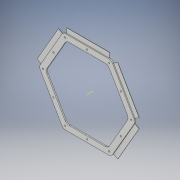
# Autodesk Inventor part: Flat Placeholder v1 - 175 - 12mm rim
Saved by Autodesk Inventor 2019 (Build 230136000, 136)
## iProperties
Created: 2021-07-14
Part Number: Flat Placeholder v1 - 175 - 12mm rim
Material: Generic
Document SubType Name: Modeling
Designer: Lix
Density: 1 g/cm^3
Appearance: Default
Author: Lix
Autodesk Inventor part; units mm, degrees
ref_plane "YZ Plane" through (0, 0, 0) normal (1, 0, 0) x (0, 1, 0)
ref_plane "XZ Plane" through (0, 0, 0) normal (0, 1, 0) x (-1, 0, 0)
ref_plane "XY Plane" through (0, 0, 0) normal (0, 0, 1) x (1, 0, 0)
sketch "Sketch1" plane through (0, 0, 0) normal (0, 0, 1) x (1, 0, 0)
  line L0 (50.5181, -87.5) -> (-50.5181, -87.5)
  line L1 (-50.5181, -87.5) -> (-101.0363, 0)
  line L2 (-101.0363, 0) -> (-50.5181, 87.5)
  line L3 (-50.5181, 87.5) -> (50.5181, 87.5)
  line L4 (50.5181, 87.5) -> (101.0363, 0)
  line L5 (101.0363, 0) -> (50.5181, -87.5)
  point P0 (0, 0)
  point P1 (0, 0)
  dimension "d0" = 175
  constraints: 12 end point, 1 coincident, 1 horizontal, 13 other
  measures "d0" distance between parallel lines of L4 L1
extrude "Extrusion1" add sketch "Sketch1" along normal blind 2
sketch "Sketch7" plane through (0, 0, 2) normal (0, 0, 1) x (1, 0, 0)
  line L0 (-50.5181, -87.5) -> (50.5181, -87.5) projected
  line L1 (50.5181, -87.5) -> (101.0363, 0) projected
  line L2 (101.0363, 0) -> (50.5181, 87.5) projected
  line L3 (50.5181, 87.5) -> (-50.5181, 87.5) projected
  line L4 (-50.5181, 87.5) -> (-101.0363, 0) projected
  line L5 (-101.0363, 0) -> (-50.5181, -87.5) projected
  line L6 (-43.5899, 75.5) -> (43.5899, 75.5)
  line L7 (43.5899, 75.5) -> (87.1799, 0)
  line L8 (87.1799, 0) -> (43.5899, -75.5)
  line L9 (43.5899, -75.5) -> (-43.5899, -75.5)
  line L10 (-43.5899, -75.5) -> (-87.1799, 0)
  line L11 (-87.1799, 0) -> (-43.5899, 75.5)
  dimension "d26" = 12
  constraints: 12 end point, 5 other
  measures "d26" distance between parallel lines of L3 L6
extrude "Extrusion6" cut sketch "Sketch7" against normal blind 7 contours L6 L7 L8 L9 L10 L11
fillet "Fillet2" radius 10 6 edges at (-87.1799, 0, 1) (-43.5899, -75.5, 1) (43.5899, -75.5, 1) (87.1799, 0, 1) (43.5899, 75.5, 1) (-43.5899, 75.5, 1)
fillet "Fillet3" radius 10 6 edges at (-50.5181, 87.5, 1) (50.5181, 87.5, 1) (101.0363, 0, 1) (50.5181, -87.5, 1) (-50.5181, -87.5, 1) (-101.0363, 0, 1)
sketch "Sketch8" plane through (0, 0, 0) normal (0, 0, -1) x (-1, 0, 0)
  line L0 (46.4767, 70.5) -> (84.2931, 5) projected
  arc A0 (84.2931, -5) -> (84.2931, 5) centre (75.6329, 0) ccw projected
  line L1 (84.2931, -5) -> (46.4767, -70.5) projected
  arc A1 (37.8164, -75.5) -> (46.4767, -70.5) centre (37.8164, -65.5) ccw projected
  line L2 (37.8164, -75.5) -> (-37.8164, -75.5) projected
  arc A2 (-46.4767, -70.5) -> (-37.8164, -75.5) centre (-37.8164, -65.5) ccw projected
  line L3 (-46.4767, -70.5) -> (-84.2931, -5) projected
  arc A3 (-84.2931, 5) -> (-84.2931, -5) centre (-75.6329, 0) ccw projected
  line L4 (-84.2931, 5) -> (-46.4767, 70.5) projected
  arc A4 (-37.8164, 75.5) -> (-46.4767, 70.5) centre (-37.8164, 65.5) ccw projected
  line L5 (-37.8164, 75.5) -> (37.8164, 75.5) projected
  arc A5 (46.4767, 70.5) -> (37.8164, 75.5) centre (37.8164, 65.5) ccw projected
  arc A6 (98.1495, -5) -> (98.1495, 5) centre (89.4893, 0) ccw projected
  line L6 (98.1495, 5) -> (53.4049, 82.5) projected
  arc A7 (53.4049, 82.5) -> (44.7446, 87.5) centre (44.7446, 77.5) ccw projected
  line L7 (44.7446, 87.5) -> (-44.7446, 87.5) projected
  arc A8 (-44.7446, 87.5) -> (-53.4049, 82.5) centre (-44.7446, 77.5) ccw projected
  line L8 (-53.4049, 82.5) -> (-98.1495, 5) projected
  arc A9 (-98.1495, 5) -> (-98.1495, -5) centre (-89.4893, 0) ccw projected
  line L9 (-98.1495, -5) -> (-53.4049, -82.5) projected
  arc A10 (-53.4049, -82.5) -> (-44.7446, -87.5) centre (-44.7446, -77.5) ccw projected
  line L10 (-44.7446, -87.5) -> (44.7446, -87.5) projected
  arc A11 (44.7446, -87.5) -> (53.4049, -82.5) centre (44.7446, -77.5) ccw projected
  line L11 (53.4049, -82.5) -> (98.1495, -5) projected
  line L12 (-53.4049, -82.5) -> (-62.0652, -87.5)
  line L13 (-62.0652, -87.5) -> (-106.8098, -10)
  line L14 (-53.4049, -82.5) -> (-98.1495, -5) projected
  line L15 (-106.8098, -10) -> (-98.1495, -5)
  line L16 (-98.1495, -5) -> (-53.4049, -82.5) projected
  line L17 (-53.4049, -82.5) -> (-98.1495, -5)
  point P0 (0, 0)
  point P1 (0, 0)
  dimension "d27" = 10
  constraints: 8 end point, 2 parallel, 2 perpendicular, 1 coincident
  measures "d27" distance between parallel lines of L9 L13
extrude "Extrusion7" add sketch "Sketch8" along normal blind 0.5
pattern_circular "Circular Pattern1" count 6 over 360 about axis through (0, 0, 0) along (0, 0, -1) of "Extrusion7"
sketch "Sketch9" plane through (0, 0, 2) normal (0, 0, 1) x (1, 0, 0)
  arc A0 (-98.1495, 5) -> (-98.1495, -5) centre (-89.4893, 0) ccw projected
  line L0 (-98.1495, -5) -> (-53.4049, -82.5) projected
  arc A1 (-53.4049, -82.5) -> (-44.7446, -87.5) centre (-44.7446, -77.5) ccw projected
  line L1 (-44.7446, -87.5) -> (44.7446, -87.5) projected
  arc A2 (44.7446, -87.5) -> (53.4049, -82.5) centre (44.7446, -77.5) ccw projected
  line L2 (53.4049, -82.5) -> (98.1495, -5) projected
  arc A3 (98.1495, -5) -> (98.1495, 5) centre (89.4893, 0) ccw projected
  line L3 (98.1495, 5) -> (53.4049, 82.5) projected
  arc A4 (53.4049, 82.5) -> (44.7446, 87.5) centre (44.7446, 77.5) ccw projected
  line L4 (44.7446, 87.5) -> (-44.7446, 87.5) projected
  arc A5 (-44.7446, 87.5) -> (-53.4049, 82.5) centre (-44.7446, 77.5) ccw projected
  line L5 (-53.4049, 82.5) -> (-98.1495, 5) projected
  line L6 (-84.2931, 5) -> (-46.4767, 70.5) projected
  arc A6 (-37.8164, 75.5) -> (-46.4767, 70.5) centre (-37.8164, 65.5) ccw projected
  line L7 (-37.8164, 75.5) -> (37.8164, 75.5) projected
  arc A7 (46.4767, 70.5) -> (37.8164, 75.5) centre (37.8164, 65.5) ccw projected
  line L8 (46.4767, 70.5) -> (84.2931, 5) projected
  arc A8 (84.2931, -5) -> (84.2931, 5) centre (75.6329, 0) ccw projected
  line L9 (84.2931, -5) -> (46.4767, -70.5) projected
  arc A9 (37.8164, -75.5) -> (46.4767, -70.5) centre (37.8164, -65.5) ccw projected
  line L10 (37.8164, -75.5) -> (-37.8164, -75.5) projected
  arc A10 (-46.4767, -70.5) -> (-37.8164, -75.5) centre (-37.8164, -65.5) ccw projected
  line L11 (-46.4767, -70.5) -> (-84.2931, -5) projected
  arc A11 (-84.2931, 5) -> (-84.2931, -5) centre (-75.6329, 0) ccw projected
  line L12 (-85.6329, 0) -> (-99.4893, 0) construction
  line L13 (-75.7772, 43.75) -> (-65.3849, 37.75) construction
  line L14 (-84.2931, 5) -> (-46.4767, 70.5) projected
  point P0 (0, 0)
  point P1 (-92.5611, 0)
  point P2 (-70.5811, 40.75)
  point P3 (-46.2805, -80.1603)
  point P4 (-70.5811, -40.75)
  point P5 (46.2805, -80.1603)
  point P6 (0, -81.5)
  point P7 (92.5611, 0)
  point P8 (70.5811, -40.75)
  point P9 (46.2805, 80.1603)
  point P10 (70.5811, 40.75)
  point P11 (-46.2805, 80.1603)
  point P12 (0, 81.5)
  dimension "d35" = 360
  constraints: 4 end point, 4 midpoint, 2 point on circle, 13 other
hole "Hole1" at (-92.5611, 0, 2) at (-70.5811, 40.75, 2) at (-46.2805, -80.1603, 2) at (-70.5811, -40.75, 2) at (46.2805, -80.1603, 2) at (0, -81.5, 2) at (92.5611, 0, 2) at (70.5811, -40.75, 2) at (46.2805, 80.1603, 2) at (70.5811, 40.75, 2) at (-46.2805, 80.1603, 2) at (0, 81.5, 2) direction (0, 0, 1) diameter 3 depth 26.75 start extended yes
sketch "Sketch10" plane through (-44.7446, -97.5, 0) normal (0, 0, 1) x (1, 0, 0)
  line L0 (0, 10) -> (89.4893, 10) projected
  line L1 (0, 0) -> (0, 10) projected
  line L2 (89.4893, 0) -> (0, 0) projected
  line L3 (89.4893, 10) -> (89.4893, 0) projected
  line L4 (-53.4049, 92.5) -> (-8.6603, 15) projected
  line L5 (-62.0652, 87.5) -> (-53.4049, 92.5) projected
  line L6 (-17.3205, 10) -> (-62.0652, 87.5) projected
  line L7 (-8.6603, 15) -> (-17.3205, 10) projected
  point P0 (44.7446, 97.5)
extrude "Extrusion8" cut sketch "Sketch10" against normal blind 10
body "Solid1"
